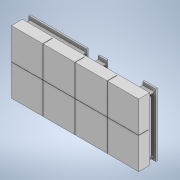
# Autodesk Inventor part: display-unit
Saved by Autodesk Inventor 2021 (Build 250183000, 183)
## iProperties
Created: 2024-04-22
Part Number: display-unit
Material: Generic
Document SubType Name: Modeling
Designer: Toby
Density: 1 g/cm^3
Appearance: Default
Author: Toby
Autodesk Inventor part; units mm, degrees
ref_plane "YZ Plane" through (0, 0, 0) normal (1, 0, 0) x (0, 1, 0)
ref_plane "XZ Plane" through (0, 0, 0) normal (0, 1, 0) x (-1, 0, 0)
ref_plane "XY Plane" through (0, 0, 0) normal (0, 0, 1) x (1, 0, 0)
sketch "Sketch1" plane through (0, 0, 0) normal (0, 0, 1) x (1, 0, 0)
  line L0 (-40.5, 20) -> (40.5, 20)
  line L1 (40.5, 20) -> (40.5, -20)
  line L2 (40.5, -20) -> (-40.5, -20)
  line L3 (-40.5, -20) -> (-40.5, 20)
  point P0 (0, 0)
  dimension "d0" = 81
  dimension "d1" = 40
  dimension "d2" = 20
  dimension "d3" = 40.5
  constraints: 8 end point, 2 parallel, 1 horizontal, 1 perpendicular
  measures "d0" distance of L0.start L0.end
  measures "d1" distance of L2.end L0.start
  measures "d2" distance from line of point (0, 0) L0
  measures "d3" distance from line of point (0, 0) L3
extrude "Extrusion1" add sketch "Sketch1" along normal blind 7
sketch "Sketch2" plane through (0, 0, 7) normal (0, 0, 1) x (1, 0, 0)
  line L0 (-40.5, 20) -> (-40.5, -20) projected
  line L1 (40.5, -20) -> (40.5, 20) projected
  line L2 (-40.5, 0.1) -> (40.5, 0.1)
  line L3 (40.5, 0.1) -> (40.5, -0.1)
  line L4 (40.5, -0.1) -> (-40.5, -0.1)
  line L5 (-40.5, -0.1) -> (-40.5, 0.1)
  line L6 (40.5, 20) -> (-40.5, 20) projected
  line L7 (-40.5, -20) -> (40.5, -20) projected
  point P0 (0, 0)
  point P1 (-40.5, -0.1)
  dimension "d6" = 19.9
  dimension "d7" = 19.9
  constraints: 8 end point, 2 parallel, 2 point on line, 1 horizontal, 1 perpendicular
  measures "d6" distance between parallel lines of L2 L6
  measures "d7" distance between parallel lines of L7 L4
extrude "Extrusion2" cut sketch "Sketch2" against normal blind 6 contours L2 L1 L4 L0
sketch "Sketch3" plane through (0, 0, 7) normal (0, 0, 1) x (1, 0, 0)
  line L0 (40.5, 20) -> (-40.5, 20) projected
  line L1 (-40.5, -20) -> (40.5, -20) projected
  line L2 (-20.6, 20) -> (-20.4, 20)
  line L3 (-20.4, 20) -> (-20.4, -20)
  line L4 (-20.4, -20) -> (-20.6, -20)
  line L5 (-20.6, -20) -> (-20.6, 20)
  line L6 (-0.1, 20) -> (0.1, 20)
  line L7 (0.1, 20) -> (0.1, -20)
  line L8 (0.1, -20) -> (-0.1, -20)
  line L9 (-0.1, -20) -> (-0.1, 20)
  line L10 (20.4, 20) -> (20.6, 20)
  line L11 (20.6, 20) -> (20.6, -20)
  line L12 (20.6, -20) -> (20.4, -20)
  line L13 (20.4, -20) -> (20.4, 20)
  line L14 (-40.5, 20) -> (-40.5, 0.1) projected
  line L15 (40.5, 0.1) -> (40.5, 20) projected
  point P0 (0, 0)
  point P1 (20.6, -20)
  dimension "d10" = 0.2
  dimension "d11" = 0.2
  dimension "d12" = 0.2
  dimension "d13" = 19.9
  dimension "d14" = 19.9
  dimension "d15" = 40.4
  dimension "d16" = 40.4
  constraints: 24 end point, 6 parallel, 6 point on line, 3 horizontal, 3 perpendicular
  measures "d10" distance between parallel lines of L3 L5
  measures "d11" distance between parallel lines of L7 L9
  measures "d12" distance between parallel lines of L13 L11
  measures "d13" distance between parallel lines of L14 L5
  measures "d14" distance between parallel lines of L15 L11
  measures "d15" distance between parallel lines of L15 L7
  measures "d16" distance between parallel lines of L14 L9
extrude "Extrusion3" cut sketch "Sketch3" against normal blind 6 contours L11 L1 L13 L0 | L7 L1 L9 L0 | L3 L1 L5 L0
sketch "Sketch4" plane through (0, 0, 0) normal (0, 0, -1) x (-1, 0, 0)
  line L0 (-39.5, 18) -> (39.5, 18)
  line L1 (39.5, 18) -> (39.5, 17.5)
  line L2 (39.5, 17.5) -> (-39.5, 17.5)
  line L3 (-39.5, 17.5) -> (-39.5, 18)
  line L4 (39.5, -17.5) -> (-39.5, -17.5)
  line L5 (-39.5, -17.5) -> (-39.5, -18)
  line L6 (-39.5, -18) -> (39.5, -18)
  line L7 (39.5, -18) -> (39.5, -17.5)
  line L8 (-40.5, 20) -> (40.5, 20) projected
  line L9 (40.5, -20) -> (-40.5, -20) projected
  line L10 (-40.5, -20) -> (-40.5, 20) projected
  line L11 (40.5, 20) -> (40.5, -20) projected
  point P0 (0, 0)
  dimension "d19" = 0.5
  dimension "d20" = 2
  dimension "d21" = 2
  dimension "d22" = 0.5
  dimension "d23" = 1
  dimension "d24" = 1
  constraints: 16 end point, 4 parallel, 2 horizontal, 2 perpendicular, 2 point on line
  measures "d19" distance between parallel lines of L2 L0
  measures "d20" distance between parallel lines of L0 L8
  measures "d21" distance between parallel lines of L9 L6
  measures "d22" distance between parallel lines of L6 L4
  measures "d23" distance between parallel lines of L10 L3
  measures "d24" distance between parallel lines of L11 L1
extrude "Extrusion4" add sketch "Sketch4" along normal blind 5 contours L0 L1 L2 L3 | L7 L6 L5 L4
sketch "Sketch5" plane through (0, 0, -5) normal (0, 0, -1) x (-1, 0, 0)
  line L0 (-40.5, -20) -> (-40.5, 20) projected
  line L1 (40.5, -20) -> (-40.5, -20) projected
  line L2 (-40.5, 20) -> (40.5, 20)
  line L3 (40.5, 20) -> (40.5, -20)
  line L4 (40.5, -20) -> (-40.5, -20)
  line L5 (-40.5, -20) -> (-40.5, 20)
  point P0 (0, 0)
  constraints: 8 end point, 2 parallel, 1 horizontal, 1 perpendicular
extrude "Extrusion5" add sketch "Sketch5" against normal blind 1
sketch "Sketch6" plane through (0, 0, -5) normal (0, 0, -1) x (-1, 0, 0)
  line L0 (-40.5, 20) -> (40.5, 20) projected
  line L1 (-3.75, 20) -> (3.75, 20)
  line L2 (3.75, 20) -> (3.75, 2)
  line L3 (3.75, 2) -> (-3.75, 2)
  line L4 (-3.75, 2) -> (-3.75, 20)
  point P0 (0, 0)
  dimension "d29" = 7.5
  dimension "d30" = 3.75
  dimension "d31" = 18
  constraints: 8 end point, 2 parallel, 1 horizontal, 1 perpendicular, 1 point on line
  measures "d29" distance of L2.end L3.end
  measures "d30" distance from line of point (0, 0) L4
  measures "d31" distance between parallel lines of L3 L0
extrude "Extrusion6" cut sketch "Sketch6" against normal blind 1
sketch "Sketch8" plane through (0, 0, -5) normal (0, 0, -1) x (-1, 0, 0)
  line L0 (-40.5, 20) -> (-40.5, -20) projected
  line L1 (-40.5, -20) -> (40.5, -20) projected
  line L2 (-40.5, 20) -> (-40.5, -20) projected
  line L3 (-40.5, -20) -> (-40.5, 20) projected
  point P0 (0, 0)
  point P1 (-35.5, 15)
  point P2 (-6.5, 17)
  point P3 (-6.5, 3)
  point P4 (6.5, 3)
  point P5 (6.5, 17)
  point P6 (-35.5, -15)
  point P7 (0, -15)
  point P8 (35.53, -15)
  point P9 (35.53, 15)
  point P10 (-40.5, 15.8)
  point P11 (-40.5, 2.8)
  dimension "d39" = 5
  dimension "d40" = 35
  dimension "d41" = 5
  dimension "d42" = 5
  dimension "d43" = 40.5
  dimension "d44" = 5
  dimension "d45" = 5
  dimension "d46" = 76.03
  dimension "d47" = 76.03
  dimension "d48" = 35
  dimension "d49" = 23
  dimension "d50" = 23
  dimension "d51" = 37
  dimension "d52" = 37
  dimension "d53" = 34
  dimension "d54" = 34
  dimension "d55" = 47
  dimension "d56" = 47
  measures "d39" distance from line of L0 point (-35.5, 15)
  measures "d40" distance from line of L1 point (-35.5, 15)
  measures "d41" distance from line of L1 point (-35.5, -15)
  measures "d42" distance from line of L2 point (-35.5, -15)
  measures "d43" distance from line of L2 point (0, -15)
  measures "d44" distance from line of L1 point (0, -15)
  measures "d45" distance from line of L1 point (35.53, -15)
  measures "d46" distance from line of L2 point (35.53, -15)
  measures "d47" distance from line of L3 point (35.53, 15)
  measures "d48" distance from line of L1 point (35.53, 15)
  measures "d49" distance from line of L1 point (-6.5, 3)
  measures "d50" distance from line of L1 point (6.5, 3)
  measures "d51" distance from line of L1 point (-6.5, 17)
  measures "d52" distance from line of L1 point (6.5, 17)
  measures "d53" distance from line of L2 point (-6.5, 17)
  measures "d54" distance from line of L2 point (-6.5, 3)
  measures "d55" distance from line of L3 point (6.5, 17)
  measures "d56" distance from line of L2 point (6.5, 3)
hole "Hole1" at (35.5, 15, -5) at (6.5, 17, -5) at (6.5, 3, -5) at (-6.5, 3, -5) at (-6.5, 17, -5) at (35.5, -15, -5) at (0, -15, -5) at (-35.53, -15, -5) at (-35.53, 15, -5) direction (0, 0, 1) diameter 2 depth 1 tip angle 118
sketch "Sketch9" plane through (-39.5, 18, 0) normal (0, 1, 0) x (1, 0, 0)
  line L0 (35.75, 5) -> (43.25, 5) projected
  line L1 (43.25, 5) -> (35.75, 5)
  line L2 (35.75, 5) -> (35.75, 0.5)
  line L3 (35.75, 0.5) -> (43.25, 0.5)
  line L4 (43.25, 0.5) -> (43.25, 5)
  line L5 (80, 0) -> (-1, 0) projected
  line L6 (35.75, 4) -> (35.75, 5) projected
  point P0 (39.5, 0)
  dimension "d64" = 0.5
  constraints: 8 end point, 2 parallel, 1 collinear, 1 horizontal, 1 perpendicular
  measures "d64" distance between parallel lines of L3 L5
extrude "Extrusion8" cut sketch "Sketch9" against normal blind 5
sketch "Sketch10" plane through (0, 0, -5) normal (0, 0, -1) x (-1, 0, 0)
  point P0 (0, 0)
sketch "Sketch11" plane through (0, 0, -5) normal (0, 0, -1) x (-1, 0, 0)
  line L0 (-3.75, 20) -> (-40.5, 20) projected
  line L1 (-40.5, 15.8) -> (-37.5, 15.8) projected
  line L2 (-37.5, 2.8) -> (-40.5, 2.8) projected
  line L3 (-40.5, -20) -> (-40.5, 20) projected
  line L4 (-37.5, 15.8) -> (-37.5, 2.8) projected
  line L5 (40.5, 20) -> (40.5, -20) projected
  line L6 (40.5, 15.8) -> (37.5, 15.8)
  line L7 (37.5, 15.8) -> (37.5, 2.8)
  line L8 (37.5, 2.8) -> (40.5, 2.8)
  line L9 (40.5, 2.8) -> (40.5, 15.8)
  line L10 (40.5, 20) -> (3.75, 20) projected
  point P0 (0, 0)
  dimension "d67" = 4.2
  dimension "d68" = 13
  dimension "d69" = 3
  dimension "d70" = 4.2
  dimension "d71" = 13
  dimension "d72" = 3
  constraints: 8 end point, 2 parallel, 1 horizontal, 1 perpendicular, 1 point on line
  measures "d67" distance between parallel lines of L0 L1
  measures "d68" distance between parallel lines of L2 L1
  measures "d69" distance between parallel lines of L3 L4
  measures "d70" distance between parallel lines of L6 L10
  measures "d71" distance between parallel lines of L6 L8
  measures "d72" distance between parallel lines of L5 L7
extrude "Extrusion9" cut sketch "Sketch11" against normal blind 1 contours L5 L8 L7 L6
sketch "Sketch12" plane through (0, 0, -5) normal (0, 0, -1) x (-1, 0, 0)
  line L0 (-40.5, 20) -> (40.5, 20) projected
  line L1 (-32.05, 20) -> (-8.95, 20)
  line L2 (-8.95, 20) -> (-8.95, 7.56)
  line L3 (-8.95, 7.56) -> (-32.05, 7.56)
  line L4 (-32.05, 7.56) -> (-32.05, 20)
  line L5 (-3.75, 2) -> (-3.75, 20) projected
  point P0 (0, 0)
  dimension "d75" = 5.2
  dimension "d76" = 12.44
  dimension "d77" = 23.1
  constraints: 8 end point, 2 parallel, 1 horizontal, 1 perpendicular, 1 point on line
  measures "d75" distance between parallel lines of L5 L2
  measures "d76" distance between parallel lines of L3 L0
  measures "d77" distance between parallel lines of L2 L4
extrude "Extrusion10" cut sketch "Sketch12" against normal blind 4.5
sketch "Sketch13" plane through (0, 0, 0) normal (0, 0, -1) x (-1, 0, 0)
  line L0 (-39.5, 16.5) -> (37.5, 16.5)
  line L1 (37.5, 16.5) -> (37.5, -16.5)
  line L2 (37.5, -16.5) -> (-39.5, -16.5)
  line L3 (-39.5, -16.5) -> (-39.5, 16.5)
  line L4 (-40.5, 20) -> (-40.5, -20) projected
  line L5 (-8.95, 17.5) -> (-32.05, 17.5) projected
  line L6 (-39.5, -17.5) -> (39.5, -17.5) projected
  line L7 (40.5, 20) -> (40.5, -20) projected
  point P0 (0, 0)
  dimension "d80" = 1
  dimension "d81" = 1
  dimension "d82" = 1
  dimension "d83" = 3
  constraints: 8 end point, 2 parallel, 1 horizontal, 1 perpendicular
  measures "d80" distance between parallel lines of L4 L3
  measures "d81" distance between parallel lines of L5 L0
  measures "d82" distance between parallel lines of L6 L2
  measures "d83" distance between parallel lines of L7 L1
extrude "Extrusion11" add sketch "Sketch13" along normal blind 2
sketch "Sketch14" plane through (0, 0, -5) normal (0, 0, -1) x (-1, 0, 0)
  line L0 (-18.1, -11.1) -> (-2.9, -11.1)
  line L1 (-2.9, -11.1) -> (-2.9, -17.3)
  line L2 (-2.9, -17.3) -> (-18.1, -17.3)
  line L3 (-18.1, -17.3) -> (-18.1, -11.1)
  line L4 (2.5, -11.1) -> (17.8, -11.1)
  line L5 (17.8, -11.1) -> (17.8, -17.3)
  line L6 (17.8, -17.3) -> (2.5, -17.3)
  line L7 (2.5, -17.3) -> (2.5, -11.1)
  line L8 (-40.5, 20) -> (-40.5, -20) projected
  line L9 (-40.5, -20) -> (40.5, -20) projected
  line L10 (-17.8, -11.4) -> (-3.2, -11.4)
  line L11 (-3.2, -11.4) -> (-3.2, -17)
  line L12 (-3.2, -17) -> (-17.8, -17)
  line L13 (-17.8, -17) -> (-17.8, -11.4)
  line L14 (2.8, -11.4) -> (17.5, -11.4)
  line L15 (17.5, -11.4) -> (17.5, -17)
  line L16 (17.5, -17) -> (2.8, -17)
  line L17 (2.8, -17) -> (2.8, -11.4)
  point P0 (0, 0)
  dimension "d86" = 22.4
  dimension "d87" = 37.6
  dimension "d88" = 43
  dimension "d89" = 58.3
  dimension "d90" = 2.7
  dimension "d91" = 6.2
  dimension "d92" = 0.3
  dimension "d93" = 0.3
  dimension "d94" = 0.3
  dimension "d95" = 0.3
  dimension "d96" = 0.3
  dimension "d97" = 0.3
  constraints: 32 end point, 8 parallel, 4 horizontal, 4 perpendicular, 4 point on line
  measures "d86" distance between parallel lines of L8 L3
  measures "d87" distance between parallel lines of L8 L1
  measures "d88" distance between parallel lines of L8 L7
  measures "d89" distance between parallel lines of L8 L5
  measures "d90" distance between parallel lines of L9 L2
  measures "d91" distance between parallel lines of L2 L0
  measures "d92" distance between parallel lines of L10 L0
  measures "d93" distance between parallel lines of L12 L2
  measures "d94" distance between parallel lines of L13 L3
  measures "d95" distance between parallel lines of L1 L11
  measures "d96" distance between parallel lines of L7 L17
  measures "d97" distance between parallel lines of L5 L15
extrude "Extrusion12" add sketch "Sketch14" along normal blind 7
sketch "Sketch15" plane through (2.9, -11.1, -5) normal (0, 1, 0) x (1, 0, 0)
  line L0 (14.9, 7) -> (0.3, 7) projected
  line L1 (14.2, 7) -> (1, 7)
  line L2 (1, 7) -> (1, 2)
  line L3 (1, 2) -> (14.2, 2)
  line L4 (14.2, 2) -> (14.2, 7)
  line L5 (-6.4, 7) -> (-19.7, 7)
  line L6 (-19.7, 7) -> (-19.7, 2)
  line L7 (-19.7, 2) -> (-6.4, 2)
  line L8 (-6.4, 2) -> (-6.4, 7)
  line L9 (-20.7, 7) -> (-5.4, 7) projected
  line L10 (13.2, 2) -> (2, 2)
  line L11 (2, 2) -> (2, 7)
  line L12 (2, 7) -> (13.2, 7)
  line L13 (13.2, 7) -> (13.2, 2)
  line L14 (-5.4, 7) -> (-20.7, 7) projected
  line L15 (-7.4, 2) -> (-18.7, 2)
  line L16 (-18.7, 2) -> (-18.7, 7)
  line L17 (-18.7, 7) -> (-7.4, 7)
  line L18 (-7.4, 7) -> (-7.4, 2)
  line L19 (15.2, 0) -> (15.2, 7) projected
  line L20 (0, 0) -> (0, 7) projected
  line L21 (-5.4, 0) -> (-5.4, 7) projected
  line L22 (-20.7, 0) -> (-20.7, 7) projected
  point P0 (-2.9, -5)
  point P1 (-18.7, 2)
  point P2 (-7.4, 7)
  point P3 (13.2, 7)
  point P4 (2, 2)
  point P5 (2, 7)
  point P6 (1, 7)
  dimension "d100" = 1
  dimension "d101" = 1
  dimension "d102" = 1
  dimension "d103" = 1
  dimension "d104" = 1
  dimension "d105" = 1
  dimension "d106" = 1
  dimension "d107" = 1
  dimension "d108" = 5
  constraints: 32 end point, 8 parallel, 6 point on line, 4 horizontal, 4 perpendicular, 1 collinear
  measures "d100" distance between parallel lines of L19 L4
  measures "d101" distance between parallel lines of L20 L2
  measures "d102" distance between parallel lines of L2 L11
  measures "d103" distance between parallel lines of L4 L13
  measures "d104" distance between parallel lines of L21 L8
  measures "d105" distance between parallel lines of L22 L6
  measures "d106" distance between parallel lines of L6 L16
  measures "d107" distance between parallel lines of L8 L18
  measures "d108" distance between parallel lines of L0 L3
extrude "Extrusion13" cut sketch "Sketch15" against normal blind 3 contours L4 L3 L13 L0 | L11 L3 L2 L0 | L8 L7 L18 L5 | L16 L7 L6 L5
body "Solid1"
